Autodesk Inventor part; units mm, degrees
(part 2 of 2)
  spline S240 degree 2 poles (41.6265, -37.0117) (41.4808, -36.8906) (41.3424, -36.5621) (41.3424, -36.3794) knots 0 0 0 1 2 2 2
  spline S241 degree 2 poles (41.3424, -36.3794) (41.3424, -36.1175) (41.6314, -35.7693) (41.9056, -35.6532) knots 0 0 0 1 2 2 2
  line L284 (41.9056, -35.6532) -> (41.9056, -35.6408)
  spline S242 degree 2 poles (41.9056, -35.6408) (41.6364, -35.5099) (41.424, -35.1369) (41.424, -34.9072) knots 0 0 0 1 2 2 2
  spline S243 degree 2 poles (41.424, -34.9072) (41.424, -34.7393) (41.5722, -34.4453) (41.7179, -34.3292) knots 0 0 0 1 2 2 2
  spline S244 degree 2 poles (41.7179, -34.3292) (41.8587, -34.2181) (42.286, -34.0847) (42.5528, -34.0847) knots 0 0 0 1 2 2 2
  spline S245 degree 2 poles (42.5528, -34.0847) (42.8343, -34.0847) (43.2542, -34.2057) (43.3901, -34.3045) knots 0 0 0 1 2 2 2
  spline S246 degree 2 poles (43.3901, -34.3045) (43.5284, -34.4033) (43.6766, -34.6899) (43.6766, -34.8554) knots 0 0 0 1 2 2 2
  spline S247 degree 2 poles (43.6766, -34.8554) (43.6766, -35.0727) (43.4247, -35.421) (43.1653, -35.542) knots 0 0 0 1 2 2 2
  line L285 (43.1653, -35.542) -> (43.1653, -35.5519)
  spline S248 degree 2 poles (43.1653, -35.5519) (43.4691, -35.6754) (43.7557, -36.0755) (43.7557, -36.3547) knots 0 0 0 1 2 2 2
  spline S249 degree 2 poles (42.9998, -36.3868) (42.9998, -36.2361) (42.8714, -36.078) (42.6639, -35.9767) knots 0 0 0 1 2 2 2
  spline S250 degree 2 poles (42.6639, -35.9767) (42.6046, -35.9496) (42.3799, -35.8631) (42.2934, -35.8261) knots 0 0 0 1 2 2 2
  spline S251 degree 2 poles (42.2934, -35.8261) (42.2144, -35.9051) (42.0884, -36.1422) (42.0884, -36.283) knots 0 0 0 1 2 2 2
  spline S252 degree 2 poles (42.0884, -36.283) (42.0884, -36.4954) (42.3601, -36.7499) (42.5799, -36.7499) knots 0 0 0 1 2 2 2
  spline S253 degree 2 poles (42.5799, -36.7499) (42.6417, -36.7499) (42.7948, -36.7103) (42.8541, -36.6708) knots 0 0 0 1 2 2 2
  spline S254 degree 2 poles (42.8541, -36.6708) (42.9208, -36.6239) (42.9998, -36.4954) (42.9998, -36.3868) knots 0 0 0 1 2 2 2
  spline S255 degree 2 poles (42.9331, -34.9443) (42.9331, -34.7887) (42.7281, -34.6034) (42.5528, -34.6034) knots 0 0 0 1 2 2 2
  spline S256 degree 2 poles (42.5528, -34.6034) (42.3848, -34.6034) (42.1798, -34.7714) (42.1798, -34.8949) knots 0 0 0 1 2 2 2
  spline S257 degree 2 poles (42.1798, -34.8949) (42.1798, -35.0159) (42.3033, -35.1666) (42.4342, -35.2283) knots 0 0 0 1 2 2 2
  spline S258 degree 2 poles (42.4342, -35.2283) (42.491, -35.258) (42.6491, -35.3197) (42.78, -35.3691) knots 0 0 0 1 2 2 2
  spline S259 degree 2 poles (42.78, -35.3691) (42.859, -35.2654) (42.9331, -35.0702) (42.9331, -34.9443) knots 0 0 0 1 2 2 2
  line L286 (48.13, -37.2019) -> (48.13, -36.0533)
  spline S260 degree 2 poles (48.13, -36.0533) (48.13, -35.8829) (48.1177, -35.6507) (48.0881, -35.5766) knots 0 0 0 1 2 2 2
  spline S261 degree 2 poles (48.0881, -35.5766) (48.0559, -35.5025) (47.9275, -35.4358) (47.8114, -35.4358) knots 0 0 0 1 2 2 2
  spline S262 degree 2 poles (47.8114, -35.4358) (47.7299, -35.4358) (47.5718, -35.5074) (47.478, -35.5741) knots 0 0 0 1 2 2 2
  line L287 (47.478, -35.5741) -> (47.478, -37.2019)
  line L288 (47.478, -37.2019) -> (46.7567, -37.2019)
  line L289 (46.7567, -37.2019) -> (46.7567, -36.0533)
  spline S263 degree 2 poles (46.7567, -36.0533) (46.7567, -35.8853) (46.7419, -35.6507) (46.7123, -35.5766) knots 0 0 0 1 2 2 2
  spline S264 degree 2 poles (46.7123, -35.5766) (46.6802, -35.5025) (46.5517, -35.4358) (46.4356, -35.4358) knots 0 0 0 1 2 2 2
  spline S265 degree 2 poles (46.4356, -35.4358) (46.3492, -35.4358) (46.1787, -35.5173) (46.0997, -35.5741) knots 0 0 0 1 2 2 2
  line L290 (46.0997, -35.5741) -> (46.0997, -37.2019)
  line L291 (46.0997, -37.2019) -> (45.3834, -37.2019)
  line L292 (45.3834, -37.2019) -> (45.3834, -34.9023)
  line L293 (45.3834, -34.9023) -> (46.0997, -34.9023)
  line L294 (46.0997, -34.9023) -> (46.0997, -35.1567)
  spline S266 degree 2 poles (46.0997, -35.1567) (46.2751, -35.0085) (46.5888, -34.8405) (46.7839, -34.8405) knots 0 0 0 1 2 2 2
  spline S267 degree 2 poles (46.7839, -34.8405) (46.9938, -34.8405) (47.3149, -35.0406) (47.3989, -35.2407) knots 0 0 0 1 2 2 2
  spline S268 degree 2 poles (47.3989, -35.2407) (47.6039, -35.048) (47.9695, -34.8405) (48.1572, -34.8405) knots 0 0 0 1 2 2 2
  spline S269 degree 2 poles (48.1572, -34.8405) (48.3178, -34.8405) (48.5722, -34.9418) (48.6586, -35.0455) knots 0 0 0 1 2 2 2
  spline S270 degree 2 poles (48.6586, -35.0455) (48.755, -35.1567) (48.8513, -35.4605) (48.8513, -35.705) knots 0 0 0 1 2 2 2
  line L295 (48.8513, -35.705) -> (48.8513, -37.2019)
  line L296 (48.8513, -37.2019) -> (48.13, -37.2019)
  line L297 (52.1265, -37.2019) -> (52.1265, -36.0533)
  spline S271 degree 2 poles (52.1265, -36.0533) (52.1265, -35.8829) (52.1142, -35.6507) (52.0845, -35.5766) knots 0 0 0 1 2 2 2
  spline S272 degree 2 poles (52.0845, -35.5766) (52.0524, -35.5025) (51.924, -35.4358) (51.8079, -35.4358) knots 0 0 0 1 2 2 2
  spline S273 degree 2 poles (51.8079, -35.4358) (51.7264, -35.4358) (51.5683, -35.5074) (51.4745, -35.5741) knots 0 0 0 1 2 2 2
  line L298 (51.4745, -35.5741) -> (51.4745, -37.2019)
  line L299 (51.4745, -37.2019) -> (50.7532, -37.2019)
  line L300 (50.7532, -37.2019) -> (50.7532, -36.0533)
  spline S274 degree 2 poles (50.7532, -36.0533) (50.7532, -35.8853) (50.7384, -35.6507) (50.7087, -35.5766) knots 0 0 0 1 2 2 2
  spline S275 degree 2 poles (50.7087, -35.5766) (50.6766, -35.5025) (50.5482, -35.4358) (50.4321, -35.4358) knots 0 0 0 1 2 2 2
  spline S276 degree 2 poles (50.4321, -35.4358) (50.3457, -35.4358) (50.1752, -35.5173) (50.0962, -35.5741) knots 0 0 0 1 2 2 2
  line L301 (50.0962, -35.5741) -> (50.0962, -37.2019)
  line L302 (50.0962, -37.2019) -> (49.3799, -37.2019)
  line L303 (49.3799, -37.2019) -> (49.3799, -34.9023)
  line L304 (49.3799, -34.9023) -> (50.0962, -34.9023)
  line L305 (50.0962, -34.9023) -> (50.0962, -35.1567)
  spline S277 degree 2 poles (50.0962, -35.1567) (50.2716, -35.0085) (50.5852, -34.8405) (50.7804, -34.8405) knots 0 0 0 1 2 2 2
  spline S278 degree 2 poles (50.7804, -34.8405) (50.9903, -34.8405) (51.3114, -35.0406) (51.3954, -35.2407) knots 0 0 0 1 2 2 2
  spline S279 degree 2 poles (51.3954, -35.2407) (51.6004, -35.048) (51.966, -34.8405) (52.1537, -34.8405) knots 0 0 0 1 2 2 2
  spline S280 degree 2 poles (52.1537, -34.8405) (52.3143, -34.8405) (52.5687, -34.9418) (52.6551, -35.0455) knots 0 0 0 1 2 2 2
  spline S281 degree 2 poles (52.6551, -35.0455) (52.7514, -35.1567) (52.8478, -35.4605) (52.8478, -35.705) knots 0 0 0 1 2 2 2
  line L306 (52.8478, -35.705) -> (52.8478, -37.2019)
  line L307 (52.8478, -37.2019) -> (52.1265, -37.2019)
  point P0 (0, 0)
  dimension "d45" = 8.7721
  dimension "d46" = 40.64
  constraints: 18 end point, 17 horizontal
  measures "d45" distance between parallel lines of L1 L0
  measures "d46" distance between parallel lines of L6 L0
extrude "Extrusion4" cut sketch "Sketch7" against normal blind 2.3813
fillet "Fillet1" radius 1.5875 9 edges at (-55.626, 0, -12.7) (-30.226, 0, -12.7) (-1.143, 0, -12.7) (29.845, 0, -12.7) (38.9043, 0, 19.05) (13.7499, 0, 19.05) (-9.3726, 0, 19.05) (-32.4951, 0, 19.05) (-55.6175, 0, 19.05)
fillet "Fillet2" radius 1.5875 4 edges at (-63.5, -3.175, 44.45) (63.5, -3.175, 44.45) (63.5, -3.175, -44.45) (-63.5, -3.175, -44.45)
equation "\"gap0\" = frontGapBetweenHoles"
equation "\"gap1\" = 0.5 * hex5mmHole + 0.5 * hex4mmHole + frontGapBetweenHoles"
equation "\"gap2\" = 0.5 * hex6mmHole + 0.5 * hex5mmHole + frontGapBetweenHoles"
equation "\"gap3\" = 0.5 * hex7mmHole + 0.5 * hex6mmHole + frontGapBetweenHoles"
equation "\"gap4\" = 0.5 * hex8mmHole + 0.5 * hex7mmHole + frontGapBetweenHoles"
equation "\"gap5\" = backGapBetweenHoles"
equation "\"gap6\" = 0.5 * hex12mmHole + 0.5 * hex10mmHole + backGapBetweenHoles"
equation "\"gap7\" = 0.5 * hex14mmHole + 0.5 * hex12mmHole + backGapBetweenHoles"
equation "\"gap8\" = 0.5 * hex17mmHole + 0.5 * hex14mmHole + backGapBetweenHoles"
equation "\"d46\" = centerLineForBackText"
equation "\"frontGapBetweenHoles\" = 7.88247"
equation "\"backGapBetweenHoles\" = 7.874"
equation "\"centerLineForFrontText\" = 8.3185"
equation "\"centerLineForBackText\" = 40.64"
body "Solid1"
